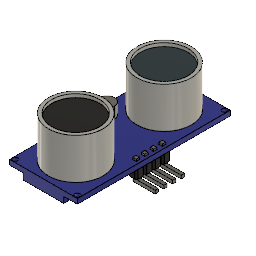
capteur_US_HCSR04 (Autodesk Fusion 360 design; units mm, degrees)
Autodesk Fusion 360 part; units mm, degrees
note: some values were not read from the file. Chosen so that the rebuilt part matches the saved one: which face or edge a step refers to.
box "BoxPrimitive1" add length 45 width 20 height 1.5 placed x (0, -1, 0) y (1, 0, 0) z (0, 0, 1) at (0, 0, 0) makes body 1
ref_plane "Plan de construction1" through (10, -22.5, 0.75) normal (1, 0, 0) x (0, 0, 1)
box "BoxPrimitive2" add length 45 width 12 height 1.8 placed x (0, -1, 0) y (-1, 0, 0) z (0, 0, -1) at (16, 0, 0) bodies 1
ref_plane "Plan de construction2" through (10, -22.5, -0.9) normal (1, 0, 0) x (0, 0, 1)
ref_plane "Plan de construction3" through (10, -22.5, -0.15) normal (0, 1, 0) x (0, 0, 1)
sketch "Esquisse3" plane through (0, 0, 1.5) normal (0, 0, 1) x (-1, 0, 0)
  line L0 (0, 45) -> (-20, 45)
  line L1 (-20, 45) -> (-20, 0)
  line L2 (-20, 0) -> (0, 0)
  line L3 (0, 0) -> (0, 45)
  circle A0 centre (-19.15, 0.85) radius 0.75
  line L4 (-10, 49.5) -> (-10, -4.5)
  circle A1 centre (-0.85, 0.85) radius 0.75
  line L5 (-22, 22.5) -> (2, 22.5)
  circle A2 centre (-19.15, 44.15) radius 0.75
  circle A3 centre (-0.85, 44.15) radius 0.75
  line L6 (-0.8, 19.3) -> (-5.2, 19.3)
  line L7 (-5.2, 19.3) -> (-5.2, 25.7)
  line L8 (-5.2, 25.7) -> (-0.8, 25.7)
  line L9 (-0.8, 25.7) -> (-0.8, 19.3)
  circle A4 centre (-3, 19.3) radius 2.2
  circle A5 centre (-3, 25.7) radius 2.2
  line L10 (-19.15, 25.88) -> (-18.15, 25.88)
  line L11 (-18.15, 25.88) -> (-18.15, 26.88)
  line L12 (-18.15, 26.88) -> (-19.15, 26.88)
  line L13 (-19.15, 26.88) -> (-19.15, 25.88)
  line L14 (-19.15, 23.32) -> (-18.15, 23.32)
  line L15 (-18.15, 23.32) -> (-18.15, 24.32)
  line L16 (-18.15, 24.32) -> (-19.15, 24.32)
  line L17 (-19.15, 24.32) -> (-19.15, 23.32)
  line L18 (-19.15, 20.76) -> (-18.15, 20.76)
  line L19 (-18.15, 20.76) -> (-18.15, 21.76)
  line L20 (-18.15, 21.76) -> (-19.15, 21.76)
  line L21 (-19.15, 21.76) -> (-19.15, 20.76)
  line L22 (-19.15, 18.2) -> (-18.15, 18.2)
  line L23 (-18.15, 18.2) -> (-18.15, 19.2)
  line L24 (-18.15, 19.2) -> (-19.15, 19.2)
  line L25 (-19.15, 19.2) -> (-19.15, 18.2)
  point P0 (-0.8, 19.3)
  point P1 (-3, 19.3)
  point P2 (13, 35)
  point P3 (-3, 25.7)
  point P4 (-19.15, 18.2)
  point P5 (-19.15, 20.76)
  point P6 (-19.15, 23.32)
  point P7 (-19.15, 25.88)
  dimension "d11" = 1.5
  dimension "d12" = 0.85
  dimension "d13" = 0.85
  dimension "d24" = 19.3
  dimension "d25" = 0.8
  dimension "d26" = 4.4
  dimension "d27" = 6.4
  dimension "d28" = 4.4
  dimension "d31" = 0.85
  dimension "d32" = 18.2
  dimension "d35" = 2.56
  dimension "d36" = 2.56
  dimension "d37" = 2.56
  dimension "d38" = 0.85
  dimension "d39" = 0.85
  dimension "d40" = 0.85
  dimension "d41" = 1
  dimension "d42" = 1
  dimension "d43" = 1
  dimension "d44" = 1
  dimension "d45" = 1
  dimension "d46" = 1
  dimension "d47" = 1
  dimension "d48" = 1
  constraint symmetric A0 L4 A1
  constraint symmetric A0 L5 A2
  constraint symmetric A1 L5 A3
  constraint horizontal L6
  constraint vertical L7
  constraint horizontal L8
  constraint vertical L9
  constraint coincident P0 L6.start
  constraint midpoint L6 P1
  constraint coincident P1 A4.centre
  constraint symmetric L5 P1 P3
  constraint symmetric L5 A4 A5
  constraint horizontal L10
  constraint vertical L11
  constraint horizontal L12
  constraint vertical L13
  constraint coincident P7 L10.start
  constraint horizontal L14
  constraint vertical L15
  constraint horizontal L16
  constraint vertical L17
  constraint coincident P6 L14.start
  constraint horizontal L18
  constraint vertical L19
  constraint horizontal L20
  constraint vertical L21
  constraint coincident P5 L18.start
  constraint horizontal L22
  constraint vertical L23
  constraint horizontal L24
  constraint vertical L25
  constraint coincident P4 L22.start
  measures "d11" diameter of A0
  measures "d12" distance of L1 A0.centre
  measures "d13" distance of L2 A0.centre
  measures "d24" distance of L2 P0
  measures "d25" distance of L3 P0
  measures "d26" distance of P0 L6.end
  measures "d27" distance of P0 L8.end
  measures "d28" diameter of A4
  measures "d31" distance of L1 P4
  measures "d32" distance of L2 P4
  measures "d35" vertical distance of P4 P5
  measures "d36" distance of P5 P6
  measures "d37" distance of P6 P7
  measures "d38" distance of L1 P5
  measures "d39" distance of L1 P6
  measures "d40" distance of L1 P7
  measures "d41" distance of P7 L10.end
  measures "d42" distance of P7 L12.end
  measures "d43" distance of P6 L14.end
  measures "d44" distance of P6 L16.end
  measures "d45" distance of P5 L18.end
  measures "d46" distance of P5 L20.end
  measures "d47" distance of P4 L22.end
  measures "d48" distance of P4 L24.end
extrude "Extrusion4" add sketch "Esquisse3" against normal blind 5.1 separate body contours L10 L11 L12 L13 | L14 L15 L16 L17 | L18 L19 L20 L21 | L22 L23 L24 L25 makes body 2 at (19.15, -23.9867, -0.2) makes body 3 at (19.15, -21.4267, -0.2) makes body 4 at (19.15, -26.5467, -0.2) makes body 5 at (19.15, -18.8667, -0.2)
extrude "Extrusion3" add sketch "Esquisse3" along normal blind 0.5 separate body contours L10 L11 L12 L13 | L14 L15 L16 L17 | L18 L19 L20 L21 | L22 L23 L24 L25 makes body 6 at (18.8167, -23.9867, 1.5) makes body 7 at (18.8167, -21.4267, 1.5) makes body 8 at (18.8167, -26.5467, 1.5) makes body 9 at (18.8167, -18.8667, 1.5)
extrude "Extrusion2" add sketch "Esquisse3" along normal blind 3.3 separate body contours L5 L7 L9 A4 | L5 L7 L9 A5 | L8 A5 | L8 A5 | L6 A4 | L6 A4 makes body 10
extrude "Extrusion1" cut sketch "Esquisse3" against normal blind 2 contours A0 | A1 | A2 | A3 bodies 1
cylinder "CylinderPrimitive1" add diameter 16 height 12 placed x (1, 0, 0) y (0, 1, 0) z (0, 0, 1) at (10, -9.5, 1.5) separate body makes body 11
hole "Perçage1" at (10, -9.5, 13.5) direction (0, 0, -1) diameter 14 depth 16 tip angle 180 bodies 11
cylinder "CylinderPrimitive2" add diameter 14 height 11 placed x (1, 0, 0) y (0, 1, 0) z (0, 0, 1) at (10, -9.503, 1.5) separate body makes body 12
mirror "Symétrie miroir1" about plane through (10, -22.5, -0.15) normal (0, 1, 0) of bodies 11 12 makes body 13 at (17.9602, -34.7035, 9.5) makes body 14 at (8.2895, -37.0841, 12.5)
combine "Combiner1" operation add target body 13 tool bodies 11 makes body 15 at (17.9602, -10.2965, 9.5)
combine "Combiner2" operation add target body 8 tool bodies 4
combine "Combiner3" operation add target body 6 tool bodies 2
combine "Combiner4" operation add target body 7 tool bodies 3
combine "Combiner5" operation add target body 9 tool bodies 5
combine "Combiner6" operation cut target body 1 tool bodies 8 6 7 9 keep tools
cylinder "CylinderPrimitive3" add diameter 1 height -1 placed x (1, 0, 0) y (0, 0, -1) z (0, 1, 0) at (18.65, -18.2, -3.6) bodies 9
cylinder "CylinderPrimitive4" add diameter 1 height -1 placed x (1, 0, 0) y (0, 0, -1) z (0, 1, 0) at (18.65, -20.76, -3.6) bodies 7
box "BoxPrimitive3" add length 0.5 width 1 height 5.6 placed x (0, 0, 1) y (0, -1, 0) z (1, 0, 0) at (19.15, -18.2, -3.6) bodies 9
extrude "Extrusion5" add 1 faces at (21.0167, -18.5333, -3.6) along direction (0, 0, -1) blind 0.5 on bodies 9 bodies 9
extrude "Extrusion6" add 1 faces at (19.15, -18.8667, -3.7667) along direction (-1, 0, 0) blind 0.5 on bodies 9 bodies 9
ref_plane "Plan de construction4" through (18.65, -19.98, -1.05) normal (0, -1, 0) x (1, 0, 0)
mirror "Symétrie miroir2" about plane through (18.65, -19.98, -1.05) normal (0, -1, 0) of bodies 9 makes body 16
ref_plane "Plan de construction5" through (18.65, -22.54, -0.8) normal (0, -1, 0) x (1, 0, 0)
mirror "Symétrie miroir3" about plane through (18.65, -22.54, -0.8) normal (0, -1, 0) of bodies 9 16 makes body 17 at (20.85, -25.88, -3.7667) makes body 18 at (20.85, -24.32, -3.7667)
sketch "Esquisse11" plane through (0, 0, 0) normal (0, 0, -1) x (1, 0, 0)
  line L0 (18.15, 19.2) -> (19.15, 19.2)
  line L1 (19.15, 19.2) -> (19.15, 18.2)
  line L2 (19.15, 18.2) -> (18.15, 18.2)
  line L3 (18.15, 18.2) -> (18.15, 19.2)
  line L4 (18.15, 21.76) -> (19.15, 21.76)
  line L5 (19.15, 21.76) -> (19.15, 20.76)
  line L6 (19.15, 20.76) -> (18.15, 20.76)
  line L7 (18.15, 20.76) -> (18.15, 21.76)
  line L8 (18.15, 24.32) -> (19.15, 24.32)
  line L9 (19.15, 24.32) -> (19.15, 23.32)
  line L10 (19.15, 23.32) -> (18.15, 23.32)
  line L11 (18.15, 23.32) -> (18.15, 24.32)
  line L12 (18.15, 26.88) -> (19.15, 26.88)
  line L13 (19.15, 26.88) -> (19.15, 25.88)
  line L14 (19.15, 25.88) -> (18.15, 25.88)
  line L15 (18.15, 25.88) -> (18.15, 26.88)
  circle A0 centre (19.15, 0.85) radius 0.75
  circle A1 centre (19.15, 44.15) radius 0.75
  line L16 (16, 45) -> (16, 0)
  line L17 (16, 0) -> (20, 0)
  line L18 (20, 0) -> (20, 45)
  line L19 (20, 45) -> (16, 45)
  line L20 (20, 24.595) -> (19.3839, 24.595)
  line L21 (20, 24.595) -> (17.45, 24.595)
  line L22 (17.45, 24.595) -> (17.45, 23.045)
  line L23 (17.45, 23.045) -> (20, 23.045)
  line L24 (20, 23.045) -> (20, 24.595)
  line L25 (17.95, 25.065) -> (19.5, 25.065)
  line L26 (19.5, 25.065) -> (19.5, 22.545)
  line L27 (19.5, 22.545) -> (17.95, 22.545)
  line L28 (17.95, 22.545) -> (17.95, 25.065)
  line L29 (17.95, 25.065) -> (17.45, 24.595)
  line L30 (19.5, 25.065) -> (20, 24.595)
  line L31 (17.45, 23.045) -> (17.95, 22.545)
  line L32 (19.5, 22.545) -> (20, 23.045)
  dimension "d69" = 2.55
  dimension "d70" = 1.55
  dimension "d71" = 2.52
  dimension "d72" = 0.5
  dimension "d73" = 0.5
  dimension "d74" = 1.55
  constraint horizontal L20
  constraint coincident L18 L20.start
  constraint horizontal L21
  constraint vertical L22
  constraint horizontal L23
  constraint vertical L24
  constraint horizontal L25
  constraint vertical L26
  constraint horizontal L27
  constraint vertical L28
  measures "d69" distance of L20.start L21.end
  measures "d70" distance of L20.start L23.end
  measures "d71" distance of L25.start L27.end
  measures "d72" horizontal distance of L22.end L27.end
  measures "d73" distance of L23 L27
  measures "d74" distance of L26.end L27.end
extrude "Extrusion7" add sketch "Esquisse11" along normal blind 2.56 separate body contours L18 L20 L21 L23 L24 L26 | L20 L21 L26 L30 | L23 L26 L32 | L20 L21 L23 L26 L28 | L20 L21 L25 L26 L28 | L23 L26 L27 L28 | L21 L28 L29 | L23 L28 L31 | L21 L22 L23 L28 makes body 19
delete_body "RemoveBody1" bodies 6
delete_body "RemoveBody2" bodies 7
delete_body "RemoveBody3" bodies 8
sketch "Esquisse12" plane through (0, 0, 12.5) normal (0, 0, 1) x (-1, 0, 0)
  circle A0 centre (-10, 9.503) radius 7
mirror "Symétrie miroir4" about plane through (18.65, -22.54, -0.8) normal (0, -1, 0) of bodies 19 makes body 20
mirror "Symétrie miroir5" about plane through (18.65, -19.98, -1.05) normal (0, -1, 0) of bodies 20 makes body 21
mirror "Symétrie miroir6" about plane through (18.65, -22.54, -0.8) normal (0, -1, 0) of bodies 21 makes body 22
named bodies: "support", "speaker1", "corps_speaker2", "speaker2", "corps_speaker1", "quartz", "pin3", "pin2", "pin4", "pin1", "plastique_pin3", "plastique_pin2", "plastique_pin1", "plastique_pin4"
